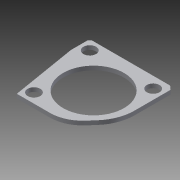
# Autodesk Inventor part: Snowblower Motor Mount
Saved by Autodesk Inventor 2013 (Build 170138000, 138)
## iProperties
Created: 2013-01-19
Part Number: Snowblower Motor Mount
Material: Aluminum 6061
Document SubType Name: Sheet Metal
Designer: actoennies
Density: 2.71 g/cm^3
Sheet Metal Rule: Default
Mass: 94.7116 g
Surface Area: 245.334 cm^2
Volume: 34.9489 cm^3
Author: actoennies
Autodesk Inventor part; units mm, degrees
ref_plane "YZ Plane" through (0, 0, 0) normal (1, 0, 0) x (0, 1, 0)
ref_plane "XZ Plane" through (0, 0, 0) normal (0, 1, 0) x (-1, 0, 0)
ref_plane "XY Plane" through (0, 0, 0) normal (0, 0, 1) x (1, 0, 0)
sketch "Sketch15" plane through (0, 3.175, 0) normal (0, 1, 0) x (1, 0, 0)
  circle A0 centre (0, 0) radius 4.953
  circle A1 centre (-6.6548, 50.2614) radius 4.953
  circle A2 centre (44.0333, 49.1637) radius 4.953
  circle A3 centre (0, 0) radius 2.54
  circle A4 centre (-6.6548, 50.2614) radius 2.54
  circle A5 centre (44.0333, 49.1637) radius 2.54
  dimension "d128" = 5.08
  dimension "d130" = 5.08
  dimension "d131" = 5.08
  measures "d128" diameter of A4
  measures "d130" diameter of A3
  measures "d131" diameter of A5
sketch "Sketch1" plane through (0, 0, 0) normal (0, 1, 0) x (-1, 0, 0)
  circle A0 centre (0, 0) radius 4.953
  circle A1 centre (0, 0) radius 2.5
  circle A2 centre (6.6548, -50.2614) radius 2.5
  circle A3 centre (6.6548, -50.2614) radius 4.953
  circle A4 centre (-44.0333, -49.1637) radius 4.953
  circle A5 centre (-44.0333, -49.1637) radius 2.5
  circle A6 centre (-22.0167, -24.5818) radius 23.8125
  line L0 (-50.309, -56.3297) -> (-48.5766, -57.8814)
  line L1 (12.6169, -57.8814) -> (14.2748, -56.0302)
  line L2 (14.2748, 0.0017) -> (5.7689, 7.62)
  line L3 (-39.1075, -0.8338) -> (-43.554, -5.7985)
  line L4 (-51.6533, -55.1257) -> (-50.309, -56.3297)
  line L5 (-48.5766, -57.8814) -> (12.6169, -57.8814)
  line L6 (14.2748, -56.0302) -> (14.2748, 0.0017)
  line L7 (-51.6533, -26.9812) -> (-51.6533, -55.1257)
  line L8 (5.7689, 7.62) -> (-20.1869, 7.62)
  arc A7 (-20.1869, 7.62) -> (-39.1075, -0.8338) centre (-20.1869, -17.78) ccw
  arc A8 (-43.554, -5.7985) -> (-51.6533, -26.9812) centre (-19.9033, -26.9812) ccw
  point P0 (-31.5358, 7.62)
  point P1 (-51.6533, -14.8414)
  dimension "d19" = 47.625
  dimension "d20" = 9.525
  dimension "d21" = 9.525
  dimension "d22" = 9.525
  dimension "d23" = 28.575
  dimension "d24" = 42.525
  dimension "d25" = 42.525
  dimension "d26" = 48.0151
  dimension "d27" = 7.62
  dimension "d28" = 7.62
  dimension "d29" = 7.62
  dimension "d30" = 7.62
  dimension "d32" = 25.4
  dimension "d33" = 31.75
  measures "d19" diameter of A6
  measures "d20" distance from line of L0 A4.centre
  measures "d21" distance from line of point (0, 0) L2
  measures "d22" distance from line of L1 A2.centre
  measures "d23" distance from line of L3 A6.centre
  measures "d24" distance from line of L2 A6.centre
  measures "d25" distance from line of L0 A6.centre
  measures "d26" distance from line of L1 A6.centre
  measures "d27" distance from line of L5 A2.centre
  measures "d28" distance from line of L6 A2.centre
  measures "d29" distance from line of L8 point (0, 0)
  measures "d30" distance from line of A5.centre L7
  measures "d32" radius of A7
  measures "d33" radius of A8
extrude "Plate3" add sketch "Sketch1" along normal blind 3.175 contours L4 L7 A8 L3 A7 L8 L2 L6 L1 L5 L0
sketch "Sketch8" plane through (0, 3.175, 0) normal (0, 1, 0) x (1, 0, 0)
  line L0 (-14.2748, -0.0017) -> (-14.2748, 56.0302) projected
  line L1 (-5.7689, -7.62) -> (-14.2748, -0.0017) projected
  line L2 (-5.7689, -7.62) -> (-14.2748, 43.18)
  dimension "d86" = 50.8
  constraints: 2 end point, 1 point on line
  measures "d86" vertical distance of L1.start L2.end
extrude "Cut2" cut sketch "Sketch8" against normal blind 3.175
sketch "Sketch9" plane through (0, 3.175, 0) normal (0, 1, 0) x (1, 0, 0)
  line L0 (20.1869, -7.62) -> (-5.7689, -7.62)
  arc A0 (20.1869, -7.62) -> (39.1075, 0.8338) centre (20.1869, 17.78) ccw
  line L1 (43.554, 5.7985) -> (39.1075, 0.8338)
  arc A1 (43.554, 5.7985) -> (51.6533, 26.9812) centre (19.9033, 26.9812) ccw
  line L2 (51.6533, 55.1257) -> (51.6533, 26.9812)
  line L3 (-14.2748, 56.0302) -> (-12.6169, 57.8814)
  circle A2 centre (0, 0) radius 4.953
  circle A3 centre (44.0333, 49.1637) radius 4.953
  line L4 (0, 0) -> (44.0333, 49.1637)
  line L5 (-5.7689, -7.62) -> (50.9928, -58.4585)
  line L6 (50.9928, -58.4585) -> (107.7358, 4.8956)
  line L7 (51.6533, 55.1257) -> (107.7358, 4.8956)
  dimension "d89" = 76.2
  measures "d89" distance of L0.end L5.end
sheet face with bend "Face5" sketch "Sketch9" thickness 3.175 toward (0, -1, 0) bend radius 3.175 relief straight relief width 3.175 relief depth 1.5875 contours A0 L1 A1 L2 L7 L6 L5 L0
bend "Bend6"
sketch "Sketch10" plane through (0, 3.175, 0) normal (0, 1, 0) x (1, 0, 0)
  line L0 (50.9928, -58.4585) -> (107.7358, 4.8956) projected
  line L1 (107.7358, 4.8956) -> (48.5766, 57.8814) projected
  circle A0 centre (92.9798, 7.456) radius 3.3782
  circle A1 centre (46.3779, -44.5755) radius 3.3782
  dimension "d95" = 6.7564
  dimension "d96" = 6.7564
  dimension "d97" = 69.85
  dimension "d98" = 7.9375
  dimension "d99" = 12.7
  dimension "d100" = 12.7
  constraints: 2 centre point
  measures "d95" diameter of A0
  measures "d96" diameter of A1
  measures "d97" distance of A1.centre A0.centre
  measures "d98" distance from line of L1 A0.centre
  measures "d99" distance from line of L0 A1.centre
  measures "d100" distance from line of L0 A0.centre
extrude "Cut3" cut sketch "Sketch10" against normal blind 3.175
sketch "Sketch11" plane through (0, 3.175, 0) normal (0, 1, 0) x (1, 0, 0)
  line L0 (-14.2748, 43.18) -> (-5.7689, -7.62)
  line L1 (-12.6169, 57.8814) -> (48.5766, 57.8814)
  line L2 (-14.2748, 56.0302) -> (-12.6169, 57.8814)
  line L3 (-14.2748, 43.18) -> (-14.2748, 56.0302)
  line L4 (48.5766, 57.8814) -> (-24.7406, 123.5477)
  line L5 (-24.7406, 123.5477) -> (-64.9877, 78.6113)
  line L6 (-64.9877, 78.6113) -> (-12.3071, 31.4281)
  dimension "d103" = 98.425
  dimension "d104" = 60.325
  measures "d103" distance of L1.end L4.end
  measures "d104" distance of L4.end L5.end
sheet face with bend "Face6" sketch "Sketch11" thickness 3.175 toward (0, -1, 0) bend radius 3.175 relief straight relief width 3.175 relief depth 1.5875
bend "Bend7"
sketch "Sketch12" plane through (0, 3.175, 0) normal (0, 1, 0) x (1, 0, 0)
  line L0 (107.7358, 4.8956) -> (-24.7406, 123.5477) projected
  line L1 (-24.7406, 123.5477) -> (-64.9877, 78.6113) projected
  circle A0 centre (-21.6351, 107.9794) radius 3.3782
  circle A1 centre (-47.0543, 79.5986) radius 3.3782
  dimension "d110" = 6.7564
  dimension "d111" = 6.7564
  dimension "d112" = 12.7
  dimension "d113" = 9.525
  dimension "d114" = 38.1
  dimension "d115" = 12.7
  constraints: 2 centre point
  measures "d110" diameter of A0
  measures "d111" diameter of A1
  measures "d112" distance from line of L1 A0.centre
  measures "d113" distance from line of L0 A0.centre
  measures "d114" distance of A1.centre A0.centre
  measures "d115" distance from line of L1 A1.centre
extrude "Cut4" cut sketch "Sketch12" against normal blind 3.175
sketch "Sketch14" plane through (0, 3.175, 0) normal (0, 1, 0) x (1, 0, 0)
  line L0 (-12.3071, 31.4281) -> (-5.7689, -7.62) projected
  line L1 (-5.7689, -7.62) -> (50.9928, -58.4585) projected
  line L2 (-6.4142, -3.7661) -> (-5.355, -2.5835)
  line L3 (-5.355, -2.5835) -> (-6.834, -1.2589)
  dimension "d124" = 1.5875
  constraints: 4 end point, 2 perpendicular, 2 point on line
  measures "d124" distance of L2.start L2.end
extrude "Cut6" cut sketch "Sketch14" against normal blind 3.175
sheet face with bend "Face7" sketch "Sketch15" thickness 3.175 toward (0, -1, 0) bend radius 3.175 relief straight relief width 3.175 relief depth 1.5875
bend "Bend8"
equation "\"d87\" = Thickness"
equation "\"d101\" = Thickness"
equation "\"d116\" = Thickness"
equation "\"d126\" = Thickness"
equation "\"d90\" = BendRadius"
equation "\"d91\" = BendReliefWidth"
equation "\"d93\" = MinimumRemnant"
equation "\"d92\" = BendReliefDepth"
equation "\"d94\" = BendRadius"
equation "\"d105\" = BendRadius"
equation "\"d106\" = BendReliefWidth"
equation "\"d108\" = MinimumRemnant"
equation "\"d107\" = BendReliefDepth"
equation "\"d109\" = BendRadius"
equation "\"d132\" = BendRadius"
equation "\"d133\" = BendReliefWidth"
equation "\"d135\" = MinimumRemnant"
equation "\"d134\" = BendReliefDepth"
equation "\"d136\" = BendRadius"
equation "\"BendRadius\" = Thickness"
equation "\"BendReliefWidth\" = Thickness"
equation "\"BendReliefDepth\" = 0.5 * Thickness"
equation "\"CornerReliefSize\" = 4 * Thickness"
equation "\"MinimumRemnant\" = 2 * Thickness"
equation "\"TransitionRadius\" = BendRadius"
equation "\"JacobiRadiusSize\" = BendRadius"
equation "\"GapSize\" = Thickness"
equation "\"d8\" = BendRadius"
equation "\"d31\" = BendRadius"
equation "\"Thickness\" = 3.175"
body "Solid2"
